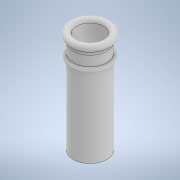
# Autodesk Inventor part: chimmney
Saved by Autodesk Inventor 2021 (Build 250183000, 183)
## iProperties
Created: 2021-08-26
Part Number: chimmney
Material: Generisch
Document SubType Name: Modeling
Designer: Tilman
Density: 1 g/cm^3
Appearance: Vorgabe
Author: Tilman
Autodesk Inventor part; units mm, degrees
ref_plane "YZ Plane" through (0, 0, 0) normal (1, 0, 0) x (0, 1, 0)
ref_plane "XZ Plane" through (0, 0, 0) normal (0, 1, 0) x (-1, 0, 0)
ref_plane "XY Plane" through (0, 0, 0) normal (0, 0, 1) x (1, 0, 0)
sketch "Skizze1" plane through (0, 0, 0) normal (0, 1, 0) x (-1, 0, 0)
  circle A0 centre (0, 0) radius 5
  dimension "d0" = 10
  constraints: 1 centre point, 1 coincident
  measures "d0" diameter of A0
extrude "Extrusion1" add sketch "Skizze1" along normal blind 25
sketch "Skizze2" plane through (0, 0, 0) normal (0, -1, 0) x (1, 0, 0)
  circle A0 centre (0, 0) radius 5 projected
  circle A1 centre (0, 0) radius 3.5
  line L0 (-3.1623, 1.5) -> (3.1623, 1.5)
  dimension "d3" = 7
  dimension "d4" = 5
  constraints: 2 end point, 2 point on circle, 1 centre point, 1 coincident, 1 horizontal
  measures "d3" diameter of A1
extrude "Extrusion2" cut sketch "Skizze2" against normal blind 10 contours A1 L0 picked at (-0.8784, -0.2211)
sketch "Skizze3" plane through (0, 0, 0) normal (0, -1, 0) x (1, 0, 0)
  circle A0 centre (0, 0) radius 5 projected
  circle A1 centre (0, 0) radius 4
  dimension "d7" = 1
  constraints: 1 centre point
  measures "d7" radial gap between concentric circles of A0 A1
extrude "Extrusion3" add sketch "Skizze3" along normal blind 5
sketch "Skizze4" plane through (0, 0, 0) normal (1, 0, 0) x (0, 1, 0)
  line L0 (-5, 5) -> (-5, -5) projected
  line L1 (25, -5) -> (25, 5) projected
  line L2 (-5, 5) -> (25, 5) projected
  arc A0 (20, 5) -> (18.5, 5) centre (19.25, 5) ccw
  arc A1 (23, 5) -> (24.2, 5.6) centre (23, 6.5) ccw
  arc A2 (25, 4) -> (24.2, 5.6) centre (25, 5) ccw
  line L3 (-10.2683, 0) -> (26.61, 0) projected
  point P0 (0, 0)
  dimension "d10" = 5
  dimension "d11" = 0.75
  dimension "d12" = 2
  dimension "d13" = 1
  dimension "d14" = 1
  constraints: 6 point on circle, 5 point on line, 3 centre point, 2 tangent, 1 line through centre
  measures "d10" distance from line of L1 A0.start
  measures "d11" radius of A0
  measures "d12" distance from line of L1 A1.start
  measures "d13" radius of A2
  measures "d14" distance of A2.start L1.end
revolve "Umdrehung1" add sketch "Skizze4" angle 360 about axis through (0, -10, 0) along (0, 1, 0) contours A0 L2 | L1 L2 A1 A2
sketch "Skizze5" plane through (0, 25, 0) normal (0, 1, 0) x (1, 0, 0)
  circle A0 centre (0, 0) radius 4 projected
extrude "Extrusion4" cut sketch "Skizze5" against normal up to surface (15 mm away)
